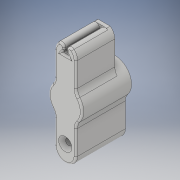
# Autodesk Inventor part: sample_hold_v2
Saved by Autodesk Inventor 2019 (Build 230136000, 136)
## iProperties
Created: 2021-12-02
Part Number: sample_hold_v2
Material: Generic
Document SubType Name: Modeling
Designer: Pokick
Density: 1 g/cm^3
Appearance: Default
Author: Pokick
Autodesk Inventor part; units mm, degrees
ref_plane "YZ Plane" through (0, 0, 0) normal (1, 0, 0) x (0, 1, 0)
ref_plane "XZ Plane" through (0, 0, 0) normal (0, 1, 0) x (-1, 0, 0)
ref_plane "XY Plane" through (0, 0, 0) normal (0, 0, 1) x (1, 0, 0)
sketch "Sketch1" plane through (0, 0, 0) normal (0, 0, 1) x (1, 0, 0)
  line L0 (0, 0) -> (0, 31) construction
  line L1 (0, 0) -> (0, -4) construction
  line L2 (0, 31) -> (0, 23.5) construction
  circle A0 centre (0, 23.5) radius 7.5 construction
  circle A1 centre (0, 0) radius 4 construction
  line L3 (4, 0) -> (4, 17.1557) construction
  line L4 (-4, 0) -> (-4, 17.1557) construction
  arc A2 (-4, 0) -> (4, 0) centre (0, 0) ccw construction
  line L5 (4, 0) -> (6, 0) construction
  line L6 (-4, 0) -> (-6, 0) construction
  arc A3 (4, 17.1557) -> (-4, 17.1557) centre (0, 23.5) ccw construction
  line L7 (6, 16.1345) -> (6, 0)
  arc A4 (-6, 0) -> (6, 0) centre (0, 0) ccw
  line L8 (-6, 0) -> (-6, 16.1345)
  arc A5 (6, 16.1345) -> (-6, 16.1345) centre (0, 23.5) ccw
  line L9 (4.1, 17.1008) -> (4.1, 0)
  arc A6 (-4.1, 0) -> (4.1, 0) centre (0, 0) ccw
  line L10 (-4.1, 0) -> (-4.1, 17.1008)
  arc A7 (4.1, 17.1008) -> (-4.1, 17.1008) centre (0, 23.5) ccw
  dimension "d0" = 31
  dimension "d1" = 4
  dimension "d2" = 7.5
  dimension "d3" = 2
  dimension "d4" = 2
  dimension "d5" = 9.5
  dimension "d6" = 0.1
  constraints: 22 end point, 20 point on circle, 8 centre point, 4 tangent, 3 parallel, 3 vertical, 2 coincident, 1 horizontal, 1 perpendicular, 1 point on line, 6 other
  measures "d0" distance of L0.start L0.end
  measures "d1" distance of L0.start L1.end
  measures "d2" distance of L0.end L2.end
  measures "d3" distance of L3.start L5.end
  measures "d4" distance of L4.start L6.end
  measures "d5" radius of A5
  measures "d6" distance between parallel lines of L3 L9
extrude "Extrusion1" add sketch "Sketch1" against normal blind 6
sketch "Sketch2" plane through (0, 0, 0) normal (0, 0, 1) x (1, 0, 0)
  line L0 (0, 0) -> (0, 31) construction
  line L1 (0, 0) -> (0, -4) construction
  line L2 (0, 31) -> (0, 23.5) construction
  circle A0 centre (0, 23.5) radius 7.5 construction
  circle A1 centre (0, 0) radius 4 construction
  line L3 (4, 0) -> (4, 17.1557) construction
  line L4 (-4, 0) -> (-4, 17.1557) construction
  arc A2 (-4, 0) -> (4, 0) centre (0, 0) ccw construction
  line L5 (4, 0) -> (6, 0) construction
  line L6 (-4, 0) -> (-6, 0) construction
  arc A3 (4, 17.1557) -> (-4, 17.1557) centre (0, 23.5) ccw construction
  line L7 (6, 16.1345) -> (6, 0)
  arc A4 (-6, 0) -> (6, 0) centre (0, 0) ccw
  line L8 (-6, 0) -> (-6, 16.1345)
  arc A5 (6, 16.1345) -> (-6, 16.1345) centre (0, 23.5) ccw
  line L9 (4.1, 17.1008) -> (4.1, 0)
  arc A6 (-4.1, 0) -> (4.1, 0) centre (0, 0) ccw
  line L10 (-4.1, 0) -> (-4.1, 17.1008)
  arc A7 (4.1, 17.1008) -> (-4.1, 17.1008) centre (0, 23.5) ccw
  line L11 (0, 0) -> (0, 3.5) construction
  circle A8 centre (0, 3.5) radius 1.75
  dimension "d9" = 31
  dimension "d10" = 4
  dimension "d11" = 7.5
  dimension "d12" = 2
  dimension "d13" = 2
  dimension "d14" = 9.5
  dimension "d15" = 0.1
  dimension "d16" = 6
  dimension "d17" = 0
  dimension "d19" = 3.5
  dimension "d21" = 3.5
  constraints: 24 end point, 20 point on circle, 9 centre point, 4 tangent, 3 coincident, 3 parallel, 3 vertical, 2 point on line, 1 horizontal, 1 perpendicular, 6 other
  measures "d9" distance of L0.start L0.end
  measures "d10" distance of L0.start L1.end
  measures "d11" distance of L0.end L2.end
  measures "d12" distance of L3.start L5.end
  measures "d13" distance of L4.start L6.end
  measures "d14" radius of A5
  measures "d15" distance between parallel lines of L3 L9
  measures "d16" distance from line of point (0, 0) L7
  measures "d17" distance from line of point (0, 0) L6
  measures "d19" distance of L11.start L11.end
  measures "d21" diameter of A8
extrude "Extrusion2" add sketch "Sketch2" along normal blind 22 contours L7 A4 L8 A5 | L9 A6 L10 A7
sketch "Sketch4" plane through (0, 0, 22) normal (0, 0, 1) x (1, 0, 0)
  line L0 (0, 0) -> (0, 53) construction
  line L1 (0, 53) -> (0, 38) construction
  line L2 (-6, 53) -> (6, 53)
  line L3 (6, 53) -> (6, 23)
  line L4 (6, 23) -> (-6, 23)
  line L5 (-6, 23) -> (-6, 53)
  line L6 (-6, 53) -> (6, 23) construction
  line L7 (6, 53) -> (-6, 23) construction
  dimension "d48" = 53
  dimension "d49" = 15
  dimension "d50" = 12
  dimension "d51" = 30
  constraints: 16 end point, 2 midpoint, 2 parallel, 1 horizontal, 1 perpendicular, 1 point on line, 1 vertical
  measures "d48" distance of L0.start L0.end
  measures "d49" distance of L0.end L1.end
  measures "d50" distance of L3.end L4.end
  measures "d51" distance of L2.end L3.end
extrude "Extrusion3" add sketch "Sketch4" against normal blind 22
fillet "Fillet1" radius 6 2 edges at (6, 53, 11) (-6, 53, 11)
fillet "Fillet2" radius 6 4 edges at (-6, 30.8655, 11) (6, 30.8655, 11) (6, 16.1345, 8) (-6, 16.1345, 8)
sketch "Sketch5" plane through (0, 0, 22) normal (0, 0, 1) x (1, 0, 0)
  line L0 (0, 0) -> (0, 53) construction
  arc A0 (6, 47) -> (-6, 47) centre (0, 47) ccw projected
  line L1 (0, 53) -> (0, 47) construction
  line L2 (0, 47) -> (0.7, 47)
  line L3 (0, 47) -> (-0.7, 47)
  line L4 (-0.7, 53) -> (0.7, 53)
  line L5 (0.7, 53) -> (0.7, 47)
  line L6 (0.7, 47) -> (-0.7, 47)
  line L7 (-0.7, 47) -> (-0.7, 53)
  line L8 (-0.7, 53) -> (0.7, 47) construction
  line L9 (0.7, 53) -> (-0.7, 47) construction
  line L10 (0, 47) -> (-2, 47)
  line L11 (0, 47) -> (2, 47)
  line L12 (2, 47) -> (0, 50)
  line L13 (-2, 47) -> (0, 50)
  dimension "d56" = 0.7
  dimension "d57" = 0.7
  dimension "d77" = 2
  dimension "d78" = 2
  constraints: 28 end point, 3 horizontal, 3 midpoint, 3 perpendicular, 2 parallel, 1 collinear, 1 point on circle, 1 vertical
  measures "d56" distance of L1.end L2.end
  measures "d57" distance of L1.end L3.end
  measures "d77" distance of L1.end L10.end
  measures "d78" distance of L1.end L11.end
extrude "Extrusion4" cut sketch "Sketch5" against normal blind 20
fillet "Fillet3" radius 2 2 edges at (0.7, 52.959, 12) (-0.7, 52.959, 12)
fillet "Fillet4" radius 1 17 edges at (1.8938, 51.7816, 22) (5.4909, 49.4188, 22) (6, 40.1554, 22) (6.3489, 31.2946, 22) (9.5, 23.5, 22) (6.3489, 15.7054, 22) (6, 6.8446, 22) (0, -6, 22) (-6, 6.8446, 22) (-6.3489, 15.7054, 22) (-9.5, 23.5, 22) (-6.3489, 31.2946, 22) (-6, 40.1554, 22) (-5.4909, 49.4188, 22) (-1.8938, 51.7816, 22) (-0.7, 49.4507, 22) (0.7, 49.4507, 22)
chamfer "Chamfer1" distance 2 angle 45 1 edges at (-1.75, 3.5, 22) measured on face at (-2.25, 3.5, 22)
fillet "Fillet5" radius 8 2 edges at (4.1, 17.1008, -3) (-4.1, 17.1008, -3)
sketch "Sketch6" plane through (0, 0, -6) normal (0, 0, -1) x (-1, 0, 0)
  arc A0 (5.8949, 18.7031) -> (-5.8949, 18.7031) centre (0, 23.5) ccw projected
  line L0 (0, 0) -> (0, 23.5) construction
  line L1 (0, 23.5) -> (0, 28.5) construction
  line L2 (0, 28.5) -> (7, 28.5)
  line L3 (7, 28.5) -> (7, 26)
  line L4 (7, 26) -> (0, 26)
  line L5 (0, 26) -> (0, 28.5)
  dimension "d66" = 5
  dimension "d67" = 7
  dimension "d68" = 2.5
  constraints: 12 end point, 2 parallel, 1 horizontal, 1 perpendicular, 1 point on line, 1 vertical
  measures "d66" distance of L0.end L1.end
  measures "d67" distance of L3.end L4.end
  measures "d68" distance of L2.end L3.end
extrude "Extrusion5" cut sketch "Sketch6" against normal blind 6
mirror "Mirror1" about plane through (0, 0, 0) normal (1, 0, 0) of "Extrusion5"
sketch "Sketch7" plane through (0, 0, 2) normal (0, 0, 1) x (1, 0, 0)
  arc A0 (6, 47) -> (-6, 47) centre (0, 47) ccw construction
  line L0 (0, 0) -> (0, 47) construction
  line L1 (0, 47) -> (2.7, 51.9513) construction
  arc A1 (4.05, 51.4269) -> (0.7, 49.9513) centre (2.7, 49.9513) ccw construction
  arc A2 (-0.7, 49.9513) -> (-4.05, 51.4269) centre (-2.7, 49.9513) ccw construction
  line L2 (-2.7, 51.9513) -> (2.7, 51.9513) construction
  line L3 (0, 51.9513) -> (5, 51.9513)
  line L4 (5, 51.9513) -> (5, 53.9513)
  line L5 (5, 53.9513) -> (0, 53.9513)
  line L6 (0, 53.9513) -> (0, 51.9513)
  line L7 (0, 51.9513) -> (-5, 51.9513)
  line L8 (-5, 51.9513) -> (-5, 53.9513)
  line L9 (-5, 53.9513) -> (0, 53.9513)
  line L10 (0, 53.9513) -> (0, 51.9513)
  dimension "d71" = 5
  dimension "d72" = 2
  dimension "d73" = 5
  dimension "d74" = 2
  constraints: 22 end point, 4 parallel, 3 horizontal, 2 perpendicular, 2 point on circle, 1 midpoint, 1 tangent, 1 vertical
  measures "d71" distance of L5.end L4.end
  measures "d72" distance of L4.end L3.end
  measures "d73" distance of L8.end L9.end
  measures "d74" distance of L7.end L8.end
extrude "Extrusion6" cut sketch "Sketch7" against normal blind 6
fillet "Fillet6" radius 1 6 edges at (0.9929, 48.5107, 21.7071) (1.85, 47.225, 22) (0.7, 48.95, 11.5) (-0.9929, 48.5107, 21.7071) (-1.85, 47.225, 22) (-0.7, 48.95, 11.5)
fillet "Fillet7" radius 1 1 edges at (0, 47, 22)
body "Solid1"
